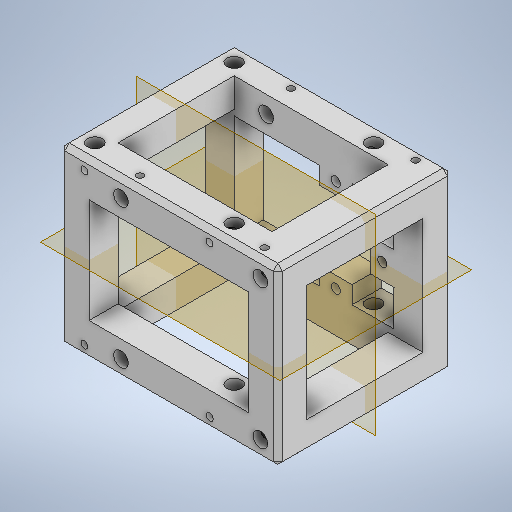
# Autodesk Inventor part: iluminator
Saved by Autodesk Inventor 2025.1 (Build 291241020, 241B)
## iProperties
Created: 2024-11-24
Part Number: iluminator
Material: Ogólny
Document SubType Name: Modeling
Designer: zychlix
Density: 1 g/cm^3
Appearance: Domyślna
Author: zychlix
Autodesk Inventor part; units mm, degrees
ref_plane "YZ Plane" through (0, 0, 0) normal (1, 0, 0) x (0, 1, 0)
ref_plane "XZ Plane" through (0, 0, 0) normal (0, 1, 0) x (-1, 0, 0)
ref_plane "XY Plane" through (0, 0, 0) normal (0, 0, 1) x (1, 0, 0)
sketch "Szkic1" plane through (0, 0, 0) normal (0, 0, 1) x (1, 0, 0)
  line L0 (86.2645, 94.401) -> (26.2645, 94.401) construction
  line L1 (26.2645, 94.401) -> (26.2645, 34.401) construction
  line L2 (26.2645, 34.401) -> (86.2645, 34.401) construction
  line L3 (86.2645, 34.401) -> (86.2645, 94.401) construction
  circle A0 centre (86.2645, 94.401) radius 3.175
  circle A1 centre (86.2645, 34.401) radius 3.175
  circle A2 centre (26.2645, 34.401) radius 3.175
  circle A3 centre (26.2645, 94.401) radius 3.175
  line L4 (93.7645, 26.901) -> (0, 26.901)
  line L5 (0, 101.901) -> (93.7645, 101.901)
  line L6 (93.7645, 101.901) -> (93.7645, 26.901)
  line L7 (12.5, 86.901) -> (81.2645, 86.901)
  line L8 (81.2645, 86.901) -> (81.2645, 41.901)
  line L9 (0, 26.901) -> (0, 101.901)
  line L10 (12.5, 86.901) -> (12.5, 41.901)
  line L11 (12.5, 41.901) -> (81.2645, 41.901)
  point P0 (0, 0)
  point P1 (56.2645, 64.401)
  point P2 (86.2645, 64.401)
  point P3 (56.2645, 94.401)
  point P4 (93.7645, 64.401)
  point P5 (0, 64.401)
  dimension "d0" = 60
  dimension "d1" = 60
  dimension "d2" = 6.35
  dimension "d8" = 75
  dimension "d39" = 7.5
  dimension "d40" = 5
  dimension "d41" = 12.5
  constraints: 24 end point, 4 centre point, 4 coincident, 4 midpoint, 3 equal radius, 3 parallel, 2 horizontal alignment, 2 perpendicular, 2 vertical, 1 horizontal, 1 point on line, 1 vertical alignment
  measures "d0" distance of L2.end L0.start
  measures "d1" distance of L1.end L2.end
  measures "d2" diameter of A0
  measures "d8" distance of L5.end L4.start
  measures "d39" distance from line of L6 L0.start
  measures "d40" distance between parallel lines of L3 L8
  measures "d41" distance from line of point (0, 64.401) L10
extrude "bryla" add sketch "Szkic1" against normal blind 75
sketch "Szkic2" plane through (0, 101.901, 0) normal (0, 1, 0) x (1, 0, 0)
  circle A0 centre (67.5, 7.5) radius 3 projected
  circle A1 centre (67.5, 67.5) radius 3 projected
  circle A2 centre (7.5, 7.5) radius 3 projected
  circle A3 centre (7.5, 67.5) radius 3 projected
  circle A4 centre (67.5, 52.5) radius 1.25 construction
  circle A5 centre (67.5, 22.5) radius 1.25 construction
  line L0 (0, 72.5) -> (2.5, 75) construction
  line L1 (0, 72.5) -> (0, 2.5) construction
  line L2 (2.5, 0) -> (0, 2.5) construction
  line L3 (2.5, 0) -> (72.5, 0) construction
  line L4 (75, 2.5) -> (72.5, 0) construction
  line L5 (75, 2.5) -> (75, 72.5) construction
  line L6 (72.5, 75) -> (75, 72.5) construction
  line L7 (72.5, 75) -> (2.5, 75) construction
  line L8 (49.43, 53.4) -> (49.43, 21.6) construction
  line L9 (49.43, 21.6) -> (25.57, 21.6) construction
  line L10 (25.57, 21.6) -> (25.57, 53.4) construction
  line L11 (25.57, 53.4) -> (49.43, 53.4) construction
  circle A6 centre (53.25, 15.725) radius 1.3 construction
  circle A7 centre (67.5, 7.5) radius 3 construction
  circle A8 centre (67.5, 67.5) radius 3 construction
  circle A9 centre (7.5, 67.5) radius 3 construction
  circle A10 centre (7.5, 7.5) radius 3 construction
  circle A11 centre (27, 64.225) radius 1.25 construction
  circle A12 centre (47.95, 64.225) radius 1.25 construction
  circle A13 centre (47.95, 11.775) radius 1.25 construction
  circle A14 centre (27, 11.775) radius 1.25 construction
  circle A15 centre (21.25, 58.875) radius 1.3 construction
  line L12 (12.5, 12.5) -> (12.5, 62.5)
  circle A16 centre (67.5, 67.5) radius 3.175
  circle A17 centre (67.5, 7.5) radius 3.175
  circle A18 centre (7.5, 7.5) radius 3.175
  circle A19 centre (7.5, 67.5) radius 3.175
  line L13 (93.7645, 0) -> (93.7645, 75) projected
  line L14 (12.5, 62.5) -> (78.7645, 62.5)
  line L15 (12.5, 12.5) -> (78.7645, 12.5)
  line L16 (78.7645, 62.5) -> (78.7645, 12.5)
  line L17 (81.2645, 0) -> (81.2645, 75) projected
  point P0 (0, 0)
  point P1 (37.5, 37.5)
  point P2 (37.5, 62.5)
  point P3 (37.5, 53.4)
  point P4 (49.43, 37.5)
  dimension "d32" = 6.35
  dimension "d37" = 12.5
  dimension "d51" = 15
  constraints: 8 end point, 4 centre point, 3 coincident, 3 equal radius, 2 horizontal, 2 midpoint, 2 vertical alignment, 1 horizontal alignment, 1 parallel
  measures "d32" diameter of A16
  measures "d37" distance between parallel lines of L1 L12
  measures "d51" distance between parallel lines of L13 L16
extrude "Wyciągnięcie proste2" cut sketch "Szkic2" against normal through all contours A0 | A1 | A2 | A3 | L12 L14 L16 L15 | A16 | A17 | A18 | A19
sketch "Szkic4" plane through (93.7645, 26.901, 0) normal (1, 0, 0) x (0, 0, -1)
  line L0 (0, 0) -> (0, 75) projected
  line L1 (0, 0) -> (75, 0) projected
  line L2 (75, 75) -> (75, 0) projected
  line L3 (0, 75) -> (75, 75) projected
  line L4 (12.5, 62.5) -> (12.5, 12.5)
  line L5 (12.5, 12.5) -> (62.5, 12.5)
  line L6 (62.5, 12.5) -> (62.5, 62.5)
  line L7 (62.5, 62.5) -> (12.5, 62.5)
  point P0 (0, -26.901)
  dimension "d17" = 12.5
  constraints: 8 end point, 3 other
  measures "d17" distance between parallel lines of L0 L4
extrude "Wyciągnięcie proste3" cut sketch "Szkic4" against normal through all contours L7 L6 L5 L4
sketch "Szkic5" plane through (0, 0, -75) normal (0, 0, -1) x (-1, 0, 0)
  line L0 (-63.2645, 39.401) -> (-49.2645, 39.401)
  line L1 (-49.2645, 39.401) -> (-49.2645, 49.401)
  line L2 (-49.2645, 49.401) -> (-63.2645, 49.401)
  line L3 (-63.2645, 49.401) -> (-63.2645, 39.401)
  line L4 (-63.2645, 79.401) -> (-49.2645, 79.401)
  line L5 (-49.2645, 79.401) -> (-49.2645, 86.901)
  line L6 (-49.2645, 86.901) -> (-63.2645, 86.901)
  line L7 (-63.2645, 86.901) -> (-63.2645, 79.401)
  line L8 (-41.2645, 57.401) -> (-31.2645, 57.401)
  line L9 (-31.2645, 57.401) -> (-31.2645, 71.401)
  line L10 (-31.2645, 71.401) -> (-41.2645, 71.401)
  line L11 (-41.2645, 71.401) -> (-41.2645, 57.401)
  line L12 (-31.2645, 39.401) -> (-81.2645, 39.401) construction
  line L13 (-31.2645, 86.901) -> (-31.2645, 39.401) construction
  line L14 (-81.2645, 86.901) -> (-12.5, 86.901) construction
  circle A0 centre (-56.2645, 44.401) radius 2
  circle A1 centre (-36.2645, 64.401) radius 2
  circle A2 centre (-56.2645, 84.401) radius 2
  circle A3 centre (-76.2645, 64.401) radius 2
  line L15 (-81.2645, 86.901) -> (-81.2645, 41.901) projected
  line L16 (-71.2645, 57.401) -> (-81.2645, 57.401)
  line L17 (-81.2645, 57.401) -> (-81.2645, 71.401)
  line L18 (-81.2645, 71.401) -> (-71.2645, 71.401)
  line L19 (-71.2645, 71.401) -> (-71.2645, 57.401)
  point P0 (0, 0)
  point P1 (-56.2645, 64.401)
  point P2 (-41.2645, 64.401)
  point P3 (-56.2645, 49.401)
  point P4 (-56.2645, 79.401)
  point P5 (-76.2645, 71.401)
  point P6 (-76.2645, 57.401)
  dimension "d20" = 15
  dimension "d21" = 15
  dimension "d22" = 15
  dimension "d23" = 14
  dimension "d24" = 4
  dimension "d27" = 360
  dimension "d29" = 20
  dimension "d42" = 15
  constraints: 32 end point, 8 parallel, 5 collinear, 5 midpoint, 5 perpendicular, 4 centre point, 4 horizontal, 3 point on line, 2 vertical alignment, 1 horizontal alignment, 9 other
  measures "d20" distance from line of L2 point (-56.264, 64.401)
  measures "d21" distance from line of L4 point (-56.264, 64.401)
  measures "d22" distance from line of point (-56.264, 64.401) L11
  measures "d23" distance of L1.end L2.end
  measures "d24" diameter of A0
  measures "d29" distance of point (-56.264, 64.401) A0.centre
  measures "d42" distance from line of point (-56.264, 64.401) L19
extrude "Wyciągnięcie proste4" add sketch "Szkic5" against normal up to surface (12.5 mm away) contours L3 L2 L1 L0 | L7 L6 L5 L4 | L18 L19 L16 L15
ref_plane "Płaszczyzna konstrukcyjna1" through (0, 64.401, 0) normal (0, 1, 0) x (1, 0, 0)
sketch "Szkic6" plane through (0, 0, 0) normal (0, 0, 1) x (1, 0, 0)
  line L0 (70.5, 7.3) -> (70.5, 507.3) construction
  line L1 (64.5, 7.3) -> (64.5, 507.3) construction
  line L2 (10.5, 0) -> (10.5, 500) construction
  line L3 (4.5, 0) -> (4.5, 500) construction
  line L4 (64.325, 101.901) -> (64.325, 86.901) projected
  circle A0 centre (64.325, 96.901) radius 1.5
  circle A1 centre (10.5, 96.901) radius 1.5
  line L5 (93.7645, 101.901) -> (0, 101.901) projected
  circle A2 centre (64.5, 31.901) radius 1.5
  circle A3 centre (10.5, 31.901) radius 1.5
  line L6 (0, 26.901) -> (93.7645, 26.901) projected
  point P0 (0, 0)
  dimension "d44" = 3
  dimension "d46" = 5
  dimension "d48" = 5
  constraints: 8 end point, 4 centre point, 4 vertical, 3 equal radius, 3 point on line, 2 horizontal alignment, 1 vertical alignment, 8 other
  measures "d44" diameter of A0
  measures "d46" distance from line of L5 A0.centre
  measures "d48" distance from line of L6 A3.centre
extrude "Wyciągnięcie proste5" cut sketch "Szkic6" against normal blind 10
sketch "Szkic9" plane through (0, 26.901, 0) normal (0, -1, 0) x (1, 0, 0)
  line L0 (89.4395, -75) -> (89.4395, 0) projected
  line L1 (83.0895, -75) -> (83.0895, 0) projected
  line L2 (29.4395, -12.5) -> (29.4395, 0) projected
  line L3 (23.0895, -12.5) -> (23.0895, 0) projected
  circle A0 centre (83.0895, -5) radius 1.5
  circle A1 centre (29.4395, -5) radius 1.5
  line L4 (83.0895, -75) -> (83.0895, 0) projected
  circle A2 centre (83.0895, -70) radius 1.5
  circle A3 centre (29.4395, -70) radius 1.5
  point P0 (0, 0)
  dimension "d52" = 3
  dimension "d53" = 5
  dimension "d57" = 5
  constraints: 4 centre point, 3 equal radius, 3 point on line, 2 horizontal alignment, 2 vertical alignment
  measures "d52" diameter of A0
  measures "d53" distance of L1.end A0.centre
  measures "d57" distance of L1.start A2.centre
extrude "Wyciągnięcie proste6" cut sketch "Szkic9" against normal blind 10
mirror "Odbij2" about plane through (0, 64.401, 0) normal (0, 1, 0) of "Wyciągnięcie proste6"
ref_plane "Płaszczyzna konstrukcyjna3" through (0, 0, -37.5) normal (0, 0, 1) x (1, 0, 0)
mirror "Odbij3" about plane through (0, 0, -37.5) normal (0, 0, 1) of "Wyciągnięcie proste5"
chamfer "Faza2" distance 2 angle 45 12 edges at (93.7645, 64.401, 0) (93.7645, 101.901, -37.5) (93.7645, 26.901, -37.5) (93.7645, 64.401, -75) (46.8822, 101.901, -75) (46.8822, 101.901, 0) (0, 101.901, -37.5) (0, 64.401, 0) (46.8822, 26.901, 0) (0, 26.901, -37.5) (0, 64.401, -75) (46.8822, 26.901, -75)
